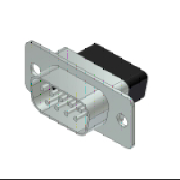
# Autodesk Inventor part: D-Sub Male 37CKT Crimp
Saved by Autodesk Inventor 2017 (Build 210142000, 142)
## iProperties
Created: 2016-02-22
Part Number: D-Sub Male 37CKT Crimp
Material: Générique
Description: Bouchon, Connecteur sous-miniature D
Document SubType Name: Modeling
Designer: Adrien MARY
Language: fr-FR
Size Designation: D-Sub Male Crimp 37CKT
Categories: <MemberInstance><Categories><Category DisplayName="Câble et faisceau" InternalName="e4a7e005-5e42-4d16-b293-125e7f0d0512" Mnemonic="CABLEANDHARNESS"><Category DisplayName="Raccords" InternalName="6f634eba-a678-4820-a31d-2c2d5ee6728e" Mnemonic="CONNECTORS"><CategoryParameter DisplayName="RefDes" InternalName="c3740e8c-60ab-4d5d-8584-52b73222f2f0" Mnemonic="REFDES"/><Category DisplayName="Fil discret" InternalName="9a3407de-09b2-4cdb-8c40-9708d5144a28" Mnemonic="DISCRETEWIRE"/></Category></Category><Category DisplayName="Type de données" InternalName="23b78d0f-2648-40c6-8793-ca6db495c9e8" Mnemonic="DATATYPE"><CategoryParameter DisplayName="AfficherNom" InternalName="05415f3d-3907-474b-a020-eb9d644f4cf3" Mnemonic="DISPLAYNAME"/><CategoryParameter DisplayName="Norme" InternalName="0c0a119c-1e12-4c84-803f-101930972f5e" Mnemonic="STANDARD"/><CategoryParameter DisplayName="Description" InternalName="13903e3d-64b1-4950-80da-f627842ea37f" Mnemonic="DESCRIPTION"/><CategoryParameter DisplayName="Désignation" InternalName="2675968c-4ce5-49e0-a4f5-552d29089031" Mnemonic="DESIGNATION"/><CategoryParameter DisplayName="Ligne par défaut" InternalName="2af9ec52-faaa-4026-b378-f9fa4afca842" Mnemonic="DEFAULTROW"/><CategoryParameter DisplayName="Nom de dossier" InternalName="3f06958e-8713-4116-9be7-ed6184ecc97b" Mnemonic="FOLDERNAME"/><CategoryParameter DisplayName="Guide révision" InternalName="45a75005-10b1-4dfc-8d6d-dfe629f0b93c" Mnemonic="REVISIONGUID"/><CategoryParameter DisplayName="NomFichier" InternalName="8b46a4cc-9585-4fed-90c3-899f57e09a73" Mnemonic="FILENAME"/><CategoryParameter DisplayName="OrgNorm" InternalName="8f5914e1-4693-403f-8ab5-d37768198c9d" Mnemonic="STDSORG"/><CategoryParameter DisplayName="Version de la famille" InternalName="914462f6-6e19-4b14-ba84-155b9680b1d0" Mnemonic="FAMILYREVISION"/><CategoryParameter DisplayName="Version standard" InternalName="91d5a463-65c2-4fde-b823-3b7fea5e8e17" Mnemonic="STANDARDREVISION"/><CategoryParameter DisplayName="Révision de membre" InternalName="a65d44b9-392f-4f4f-857b-e4b3d54996fe" Mnemonic="MEMBERREVISION"/><CategoryParameter DisplayName="DélimiterFormat" InternalName="bc51e27b-3422-4e78-93ef-cec197ddf230" Mnemonic="CLIPFORMAT"/><CategoryParameter DisplayName="Fabricant" InternalName="cd6c7a72-a28a-4e50-99a9-2c7f4e13e5ad" Mnemonic="MANUFACTURER"/><CategoryParameter DisplayName="NomInterne" InternalName="cf1d0246-76d9-4b4a-8305-fa0409afb5c1" Mnemonic="INTERNALNAME"/><CategoryParameter DisplayName="Métrique" InternalName="e2385c5b-1ea4-4823-96a8-8de651266ec3" Mnemonic="ISMETRIC"/><Category DisplayName="Pièce" InternalName="c0e0b642-3bcb-4cc8-9e80-f96d35c4afa4" Mnemonic="PART"><CategoryParameter DisplayName="Numéro de pièce" InternalName="016b6077-bfbe-49bd-92c9-d8d59c39c941" Mnemonic="PARTNUMBER"/><CategoryParameter DisplayName="Numéro de stock" InternalName="4dba7c1c-e26c-444e-836c-b08b433409a8" Mnemonic="STOCKNUMBER"/><CategoryParameter DisplayName="Clé matière" InternalName="5c9a8adb-dd2b-4535-b97f-0a94a95fe41f" Mnemonic="MATERIALKEY"/><CategoryParameter DisplayName="Matière" InternalName="818a152a-d3c3-49ca-80ee-df7d91421b8e" Mnemonic="MATERIAL"/></Category></Category></Categories><FamilyTemplate Id="D-Sub Male Crimp"><FamilyTemplateParameters><FamilyTemplateParameter ObjectType="kUserParameterObject" ValueType="xs:double" Id="1" ObjectReferenceKey="DimA"/><FamilyTemplateParameter ObjectType="kUserParameterObject" ValueType="xs:double" Id="2" ObjectReferenceKey="DimB"/><FamilyTemplateParameter ObjectType="kUserParameterObject" ValueType="xs:double" Id="3" ObjectReferenceKey="DimC"/><FamilyTemplateParameter ObjectType="kUserParameterObject" ValueType="xs:double" Id="4" ObjectReferenceKey="DimD"/><FamilyTemplateParameter ObjectType="kUserParameterObject" ValueType="xs:double" Id="5" ObjectReferenceKey="DimE"/><FamilyTemplateParameter ObjectType="kUserParameterObject" ValueType="xs:double" Id="6" ObjectReferenceKey="Holes_R1"/><FamilyTemplateParameter ObjectType="kUserParameterObject" ValueType="xs:double" Id="7" ObjectReferenceKey="Holes_R2"/><FamilyTemplateParameter ObjectType="kUserParameterObject" ValueType="xs:double" Id="8" ObjectReferenceKey="P10C"/><FamilyTemplateParameter ObjectType="kUserParameterObject" ValueType="xs:double" Id="9" ObjectReferenceKey="P10R"/><FamilyTemplateParameter ObjectType="kUserParameterObject" ValueType="xs:double" Id="10" ObjectReferenceKey="P11C"/><FamilyTemplateParameter ObjectType="kUserParameterObject" ValueType="xs:double" Id="11" ObjectReferenceKey="P11R"/><FamilyTemplateParameter ObjectType="kUserParameterObject" ValueType="xs:double" Id="12" ObjectReferenceKey="P12C"/><FamilyTemplateParameter ObjectType="kUserParameterObject" ValueType="xs:double" Id="13" ObjectReferenceKey="P12R"/><FamilyTemplateParameter ObjectType="kUserParameterObject" ValueType="xs:double" Id="14" ObjectReferenceKey="P13C"/><FamilyTemplateParameter ObjectType="kUserParameterObject" ValueType="xs:double" Id="15" ObjectReferenceKey="P13R"/><FamilyTemplateParameter ObjectType="kUserParameterObject" ValueType="xs:double" Id="16" ObjectReferenceKey="P14C"/><FamilyTemplateParameter ObjectType="kUserParameterObject" ValueType="xs:double" Id="17" ObjectReferenceKey="P14R"/><FamilyTemplateParameter ObjectType="kUserParameterObject" ValueType="xs:double" Id="18" ObjectReferenceKey="P15C"/><FamilyTemplateParameter ObjectType="kUserParameterObject" ValueType="xs:double" Id="19" ObjectReferenceKey="P15R"/><FamilyTemplateParameter ObjectType="kUserParameterObject" ValueType="xs:double" Id="20" ObjectReferenceKey="P16C"/><FamilyTemplateParameter ObjectType="kUserParameterObject" ValueType="xs:double" Id="21" ObjectReferenceKey="P16R"/><FamilyTemplateParameter ObjectType="kUserParameterObject" ValueType="xs:double" Id="22" ObjectReferenceKey="P17C"/><FamilyTemplateParameter ObjectType="kUserParameterObject" ValueType="xs:double" Id="23" ObjectReferenceKey="P17R"/><FamilyTemplateParameter ObjectType="kUserParameterObject" ValueType="xs:double" Id="24" ObjectReferenceKey="P18C"/><FamilyTemplateParameter ObjectType="kUserParameterObject" ValueType="xs:double" Id="25" ObjectReferenceKey="P18R"/><FamilyTemplateParameter ObjectType="kUserParameterObject" ValueType="xs:double" Id="26" ObjectReferenceKey="P19C"/><FamilyTemplateParameter ObjectType="kUserParameterObject" ValueType="xs:double" Id="27" ObjectReferenceKey="P19R"/><FamilyTemplateParameter ObjectType="kUserParameterObject" ValueType="xs:double" Id="28" ObjectReferenceKey="P20C"/><FamilyTemplateParameter ObjectType="kUserParameterObject" ValueType="xs:double" Id="29" ObjectReferenceKey="P20R"/><FamilyTemplateParameter ObjectType="kUserParameterObject" ValueType="xs:double" Id="30" ObjectReferenceKey="P21C"/><FamilyTemplateParameter ObjectType="kUserParameterObject" ValueType="xs:double" Id="31" ObjectReferenceKey="P21R"/><FamilyTemplateParameter ObjectType="kUserParameterObject" ValueType="xs:double" Id="32" ObjectReferenceKey="P22C"/><FamilyTemplateParameter ObjectType="kUserParameterObject" ValueType="xs:double" Id="33" ObjectReferenceKey="P22R"/><FamilyTemplateParameter ObjectType="kUserParameterObject" ValueType="xs:double" Id="34" ObjectReferenceKey="P23C"/><FamilyTemplateParameter ObjectType="kUserParameterObject" ValueType="xs:double" Id="35" ObjectReferenceKey="P23R"/><FamilyTemplateParameter ObjectType="kUserParameterObject" ValueType="xs:double" Id="36" ObjectReferenceKey="P24C"/><FamilyTemplateParameter ObjectType="kUserParameterObject" ValueType="xs:double" Id="37" ObjectReferenceKey="P24R"/><FamilyTemplateParameter ObjectType="kUserParameterObject" ValueType="xs:double" Id="38" ObjectReferenceKey="P25C"/><FamilyTemplateParameter ObjectType="kUserParameterObject" ValueType="xs:double" Id="39" ObjectReferenceKey="P25R"/><FamilyTemplateParameter ObjectType="kUserParameterObject" ValueType="xs:double" Id="40" ObjectReferenceKey="P26C"/><FamilyTemplateParameter ObjectType="kUserParameterObject" ValueType="xs:double" Id="41" ObjectReferenceKey="P26R"/><FamilyTemplateParameter ObjectType="kUserParameterObject" ValueType="xs:double" Id="42" ObjectReferenceKey="P27C"/><FamilyTemplateParameter ObjectType="kUserParameterObject" ValueType="xs:double" Id="43" ObjectReferenceKey="P27R"/><FamilyTemplateParameter ObjectType="kUserParameterObject" ValueType="xs:double" Id="44" ObjectReferenceKey="P28C"/><FamilyTemplateParameter ObjectType="kUserParameterObject" ValueType="xs:double" Id="45" ObjectReferenceKey="P28R"/><FamilyTemplateParameter ObjectType="kUserParameterObject" ValueType="xs:double" Id="46" ObjectReferenceKey="P29C"/><FamilyTemplateParameter ObjectType="kUserParameterObject" ValueType="xs:double" Id="47" ObjectReferenceKey="P29R"/><FamilyTemplateParameter ObjectType="kUserParameterObject" ValueType="xs:double" Id="48" ObjectReferenceKey="P30C"/><FamilyTemplateParameter ObjectType="kUserParameterObject" ValueType="xs:double" Id="49" ObjectReferenceKey="P30R"/><FamilyTemplateParameter ObjectType="kUserParameterObject" ValueType="xs:double" Id="50" ObjectReferenceKey="P31C"/><FamilyTemplateParameter ObjectType="kUserParameterObject" ValueType="xs:double" Id="51" ObjectReferenceKey="P31R"/><FamilyTemplateParameter ObjectType="kUserParameterObject" ValueType="xs:double" Id="52" ObjectReferenceKey="P32C"/><FamilyTemplateParameter ObjectType="kUserParameterObject" ValueType="xs:double" Id="53" ObjectReferenceKey="P32R"/><FamilyTemplateParameter ObjectType="kUserParameterObject" ValueType="xs:double" Id="54" ObjectReferenceKey="P33C"/><FamilyTemplateParameter ObjectType="kUserParameterObject" ValueType="xs:double" Id="55" ObjectReferenceKey="P33R"/><FamilyTemplateParameter ObjectType="kUserParameterObject" ValueType="xs:double" Id="56" ObjectReferenceKey="P34C"/><FamilyTemplateParameter ObjectType="kUserParameterObject" ValueType="xs:double" Id="57" ObjectReferenceKey="P34R"/><FamilyTemplateParameter ObjectType="kUserParameterObject" ValueType="xs:double" Id="58" ObjectReferenceKey="P35C"/><FamilyTemplateParameter ObjectType="kUserParameterObject" ValueType="xs:double" Id="59" ObjectReferenceKey="P35R"/><FamilyTemplateParameter ObjectType="kUserParameterObject" ValueType="xs:double" Id="60" ObjectReferenceKey="P36C"/><FamilyTemplateParameter ObjectType="kUserParameterObject" ValueType="xs:double" Id="61" ObjectReferenceKey="P36R"/><FamilyTemplateParameter ObjectType="kUserParameterObject" ValueType="xs:double" Id="62" ObjectReferenceKey="P37C"/><FamilyTemplateParameter ObjectType="kUserParameterObject" ValueType="xs:double" Id="63" ObjectReferenceKey="P6C"/><FamilyTemplateParameter ObjectType="kUserParameterObject" ValueType="xs:double" Id="64" ObjectReferenceKey="P6R"/><FamilyTemplateParameter ObjectType="kUserParameterObject" ValueType="xs:double" Id="65" ObjectReferenceKey="P7C"/><FamilyTemplateParameter ObjectType="kUserParameterObject" ValueType="xs:double" Id="66" ObjectReferenceKey="P7R"/><FamilyTemplateParameter ObjectType="kUserParameterObject" ValueType="xs:double" Id="67" ObjectReferenceKey="P8C"/><FamilyTemplateParameter ObjectType="kUserParameterObject" ValueType="xs:double" Id="68" ObjectReferenceKey="P8R"/><FamilyTemplateParameter ObjectType="kUserParameterObject" ValueType="xs:double" Id="69" ObjectReferenceKey="P9C"/><FamilyTemplateParameter ObjectType="kUserParameterObject" ValueType="xs:double" Id="70" ObjectReferenceKey="P9R"/><FamilyTemplateParameter ObjectType="kPropertyObject" ValueType="xs:string" Id="100" ObjectReferenceKey="{32853F0F-3444-11d1-9E93-0060B03C1CA6}" SubObjectId="52"/><FamilyTemplateParameter ObjectType="kPropertyObject" ValueType="xs:string" Id="105" ObjectReferenceKey="{32853F0F-3444-11d1-9E93-0060B03C1CA6}" SubObjectId="5"/><FamilyTemplateParameter ObjectType="kPartComponentDefinitionObject" ValueType="xs:string" Id="110" SubObjectId="Material"/><FamilyTemplateParameter ObjectType="kPartFeatureObject" ValueType="xs:boolean" Id="200" ObjectReferenceKey="10020000100000005cbc0200000000008000000000000000" SubObjectId="Suppressed"/><FamilyTemplateParameter ObjectType="kPartFeatureObject" ValueType="xs:boolean" Id="201" ObjectReferenceKey="100200001000000077bc0200000000008000000000000000" SubObjectId="Suppressed"/><FamilyTemplateParameter ObjectType="kPartFeatureObject" ValueType="xs:boolean" Id="202" ObjectReferenceKey="10020000100000007abc0200000000008000000000000000" SubObjectId="Suppressed"/><FamilyTemplateParameter ObjectType="kPartFeatureObject" ValueType="xs:boolean" Id="203" ObjectReferenceKey="10020000100000007dbc0200000000008000000000000000" SubObjectId="Suppressed"/><FamilyTemplateParameter ObjectType="kPartFeatureObject" ValueType="xs:boolean" Id="204" ObjectReferenceKey="100200001000000080bc0200000000008000000000000000" SubObjectId="Suppressed"/><FamilyTemplateParameter ObjectType="kPartFeatureObject" ValueType="xs:boolean" Id="205" ObjectReferenceKey="100200001000000083bc0200000000008000000000000000" SubObjectId="Suppressed"/><FamilyTemplateParameter ObjectType="kPartFeatureObject" ValueType="xs:boolean" Id="206" ObjectReferenceKey="100200001000000086bc0200000000008000000000000000" SubObjectId="Suppressed"/><FamilyTemplateParameter ObjectType="kPartFeatureObject" ValueType="xs:boolean" Id="207" ObjectReferenceKey="100200001000000089bc0200000000008000000000000000" SubObjectId="Suppressed"/><FamilyTemplateParameter ObjectType="kPartFeatureObject" ValueType="xs:boolean" Id="208" ObjectReferenceKey="10020000100000008cbc0200000000008000000000000000" SubObjectId="Suppressed"/><FamilyTemplateParameter ObjectType="kPartFeatureObject" ValueType="xs:boolean" Id="209" ObjectReferenceKey="10020000100000008fbc0200000000008000000000000000" SubObjectId="Suppressed"/><FamilyTemplateParameter ObjectType="kPartFeatureObject" ValueType="xs:boolean" Id="210" ObjectReferenceKey="100200001000000092bc0200000000008000000000000000" SubObjectId="Suppressed"/><FamilyTemplateParameter ObjectType="kPartFeatureObject" ValueType="xs:boolean" Id="211" ObjectReferenceKey="10020000100000005fbc0200000000008000000000000000" SubObjectId="Suppressed"/><FamilyTemplateParameter ObjectType="kPartFeatureObject" ValueType="xs:boolean" Id="212" ObjectReferenceKey="100200001000000095bc0200000000008000000000000000" SubObjectId="Suppressed"/><FamilyTemplateParameter ObjectType="kPartFeatureObject" ValueType="xs:boolean" Id="213" ObjectReferenceKey="100200001000000098bc0200000000008000000000000000" SubObjectId="Suppressed"/><FamilyTemplateParameter ObjectType="kPartFeatureObject" ValueType="xs:boolean" Id="214" ObjectReferenceKey="10020000100000009bbc0200000000008000000000000000" SubObjectId="Suppressed"/><FamilyTemplateParameter ObjectType="kPartFeatureObject" ValueType="xs:boolean" Id="215" ObjectReferenceKey="10020000100000009ebc0200000000008000000000000000" SubObjectId="Suppressed"/><FamilyTemplateParameter ObjectType="kPartFeatureObject" ValueType="xs:boolean" Id="216" ObjectReferenceKey="1002000010000000a1bc0200000000008000000000000000" SubObjectId="Suppressed"/><FamilyTemplateParameter ObjectType="kPartFeatureObject" ValueType="xs:boolean" Id="217" ObjectReferenceKey="1002000010000000a4bc0200000000008000000000000000" SubObjectId="Suppressed"/><FamilyTemplateParameter ObjectType="kPartFeatureObject" ValueType="xs:boolean" Id="218" ObjectReferenceKey="1002000010000000a7bc0200000000008000000000000000" SubObjectId="Suppressed"/><FamilyTemplateParameter ObjectType="kPartFeatureObject" ValueType="xs:boolean" Id="219" ObjectReferenceKey="1002000010000000aabc0200000000008000000000000000" SubObjectId="Suppressed"/><FamilyTemplateParameter ObjectType="kPartFeatureObject" ValueType="xs:boolean" Id="220" ObjectReferenceKey="1002000010000000adbc0200000000008000000000000000" SubObjectId="Suppressed"/><FamilyTemplateParameter ObjectType="kPartFeatureObject" ValueType="xs:boolean" Id="221" ObjectReferenceKey="1002000010000000b0bc0200000000008000000000000000" SubObjectId="Suppressed"/><FamilyTemplateParameter ObjectType="kPartFeatureObject" ValueType="xs:boolean" Id="222" ObjectReferenceKey="100200001000000062bc0200000000008000000000000000" SubObjectId="Suppressed"/><FamilyTemplateParameter ObjectType="kPartFeatureObject" ValueType="xs:boolean" Id="223" ObjectReferenceKey="1002000010000000b3bc0200000000008000000000000000" SubObjectId="Suppressed"/><FamilyTemplateParameter ObjectType="kPartFeatureObject" ValueType="xs:boolean" Id="224" ObjectReferenceKey="1002000010000000b6bc0200000000008000000000000000" SubObjectId="Suppressed"/><FamilyTemplateParameter ObjectType="kPartFeatureObject" ValueType="xs:boolean" Id="225" ObjectReferenceKey="1002000010000000b9bc0200000000008000000000000000" SubObjectId="Suppressed"/><FamilyTemplateParameter ObjectType="kPartFeatureObject" ValueType="xs:boolean" Id="226" ObjectReferenceKey="1002000010000000bcbc0200000000008000000000000000" SubObjectId="Suppressed"/><FamilyTemplateParameter ObjectType="kPartFeatureObject" ValueType="xs:boolean" Id="227" ObjectReferenceKey="1002000010000000bfbc0200000000008000000000000000" SubObjectId="Suppressed"/><FamilyTemplateParameter ObjectType="kPartFeatureObject" ValueType="xs:boolean" Id="228" ObjectReferenceKey="1002000010000000c2bc0200000000008000000000000000" SubObjectId="Suppressed"/><FamilyTemplateParameter ObjectType="kPartFeatureObject" ValueType="xs:boolean" Id="229" ObjectReferenceKey="1002000010000000c5bc0200000000008000000000000000" SubObjectId="Suppressed"/><FamilyTemplateParameter ObjectType="kPartFeatureObject" ValueType="xs:boolean" Id="230" ObjectReferenceKey="1002000010000000c8bc0200000000008000000000000000" SubObjectId="Suppressed"/><FamilyTemplateParameter ObjectType="kPartFeatureObject" ValueType="xs:boolean" Id="231" ObjectReferenceKey="100200001000000065bc0200000000008000000000000000" SubObjectId="Suppressed"/><FamilyTemplateParameter ObjectType="kPartFeatureObject" ValueType="xs:boolean" Id="232" ObjectReferenceKey="100200001000000068bc0200000000008000000000000000" SubObjectId="Suppressed"/><FamilyTemplateParameter ObjectType="kPartFeatureObject" ValueType="xs:boolean" Id="233" ObjectReferenceKey="10020000100000006bbc0200000000008000000000000000" SubObjectId="Suppressed"/><FamilyTemplateParameter ObjectType="kPartFeatureObject" ValueType="xs:boolean" Id="234" ObjectReferenceKey="10020000100000006ebc0200000000008000000000000000" SubObjectId="Suppressed"/><FamilyTemplateParameter ObjectType="kPartFeatureObject" ValueType="xs:boolean" Id="235" ObjectReferenceKey="100200001000000071bc0200000000008000000000000000" SubObjectId="Suppressed"/><FamilyTemplateParameter ObjectType="kPartFeatureObject" ValueType="xs:boolean" Id="236" ObjectReferenceKey="100200001000000074bc0200000000008000000000000000" SubObjectId="Suppressed"/></FamilyTemplateParameters></FamilyTemplate><CategoryParameterMap><ParamToTemplateMap><ParamToTemplate CategoryParameter="//CategoryParameter[@InternalName='05415f3d-3907-474b-a020-eb9d644f4cf3']" ConstantValue="D-Sub Male Crimp"/><ParamToTemplate CategoryParameter="//CategoryParameter[@InternalName='0c0a119c-1e12-4c84-803f-101930972f5e']" TemplateParameter="102"/><ParamToTemplate CategoryParameter="//CategoryParameter[@InternalName='13903e3d-64b1-4950-80da-f627842ea37f']" ConstantValue="Plug, Subminiature D Connector"/><ParamToTemplate CategoryParameter="//CategoryParameter[@InternalName='2af9ec52-faaa-4026-b378-f9fa4afca842']" ConstantValue="1"/><ParamToTemplate CategoryParameter="//CategoryParameter[@InternalName='3f06958e-8713-4116-9be7-ed6184ecc97b']" ConstantValue="D-Sub Male Crimp"/><ParamToTemplate CategoryParameter="//CategoryParameter[@InternalName='45a75005-10b1-4dfc-8d6d-dfe629f0b93c']" ConstantValue="6bfec97e-a90e-497f-8d9f-e40cc73ef834"/><ParamToTemplate CategoryParameter="//CategoryParameter[@InternalName='8f5914e1-4693-403f-8ab5-d37768198c9d']" TemplateParameter="101"/><ParamToTemplate CategoryParameter="//CategoryParameter[@InternalName='914462f6-6e19-4b14-ba84-155b9680b1d0']" ConstantValue="11"/><ParamToTemplate CategoryParameter="//CategoryParameter[@InternalName='91d5a463-65c2-4fde-b823-3b7fea5e8e17']" TemplateParameter="103"/><ParamToTemplate CategoryParameter="//CategoryParameter[@InternalName='bc51e27b-3422-4e78-93ef-cec197ddf230']" ConstantValue="CF_INVENTOR.STDPARTS"/><ParamToTemplate CategoryParameter="//CategoryParameter[@InternalName='cd6c7a72-a28a-4e50-99a9-2c7f4e13e5ad']" TemplateParameter="104"/><ParamToTemplate CategoryParameter="//CategoryParameter[@InternalName='cf1d0246-76d9-4b4a-8305-fa0409afb5c1']" ConstantValue="1b68272e-2c5e-46fd-a1a0-13114f04d71e"/><ParamToTemplate CategoryParameter="//CategoryParameter[@InternalName='e2385c5b-1ea4-4823-96a8-8de651266ec3']" ConstantValue="false"/><ParamToTemplate CategoryParameter="//CategoryParameter[@InternalName='8b46a4cc-9585-4fed-90c3-899f57e09a73']" ConstantValue="D-Sub Male Crimp 37CKT"/><ParamToTemplate CategoryParameter="//CategoryParameter[@InternalName='a65d44b9-392f-4f4f-857b-e4b3d54996fe']" ConstantValue="05c4e255-4499-4a76-b96a-0caab7a32f8d"/><ParamToTemplate CategoryParameter="//CategoryParameter[@InternalName='2675968c-4ce5-49e0-a4f5-552d29089031']" TemplateParameter="100"/><ParamToTemplate CategoryParameter="//CategoryParameter[@InternalName='818a152a-d3c3-49ca-80ee-df7d91421b8e']" TemplateParameter="110"/><ParamToTemplate CategoryParameter="//CategoryParameter[@InternalName='016b6077-bfbe-49bd-92c9-d8d59c39c941']" TemplateParameter="105"/></ParamToTemplateMap></CategoryParameterMap></MemberInstance>
Mass: 4.69725 g
Surface Area: 80.6213 cm^2
Volume: 4.69725 cm^3
Density: 1 g/cm^3
Appearance: Par défaut
GlobalPropertyList: <PropertyList/>
IsCustomPart: 0
Author: Adrien MARY
Autodesk Inventor part; units mm, degrees
ref_plane "YZ Plane" through (0, 0, 0) normal (1, 0, 0) x (0, 1, 0)
ref_plane "XZ Plane" through (0, 0, 0) normal (0, 1, 0) x (-1, 0, 0)
ref_plane "XY Plane" through (0, 0, 0) normal (0, 0, 1) x (1, 0, 0)
sketch "Sketch1" plane through (0, 0, 0) normal (0, 0, 1) x (1, 0, 0)
  circle A0 centre (-31.75, 0) radius 1.524
  circle A1 centre (31.75, 0) radius 1.524
  arc A2 (-33.0835, 6.2992) -> (-34.6583, 4.7244) centre (-33.0835, 4.7244) ccw
  line L0 (-34.6583, 4.7244) -> (-34.6583, -4.7244)
  arc A3 (-34.6583, -4.7244) -> (-33.0835, -6.2992) centre (-33.0835, -4.7244) ccw
  line L1 (-33.0835, -6.2992) -> (33.0835, -6.2992)
  arc A4 (33.0835, -6.2992) -> (34.6583, -4.7244) centre (33.0835, -4.7244) ccw
  line L2 (34.6583, -4.7244) -> (34.6583, 4.7244)
  arc A5 (34.6583, 4.7244) -> (33.0835, 6.2992) centre (33.0835, 4.7244) ccw
  line L3 (33.0835, 6.2992) -> (-33.0835, 6.2992)
  line L4 (0, 6.2992) -> (0, -6.2992) construction
  line L5 (-31.75, 0) -> (31.75, 0) construction
  line L6 (34.6583, 4.7244) -> (33.0835, 4.7244) construction
  line L7 (33.0835, 4.7244) -> (33.0835, 6.2992) construction
  line L8 (34.6583, -4.7244) -> (33.0835, -4.7244) construction
  line L9 (33.0835, -4.7244) -> (33.0835, -6.2992) construction
  line L10 (-33.0835, 6.2992) -> (-33.0835, 4.7244) construction
  line L11 (-33.0835, 4.7244) -> (-34.6583, 4.7244) construction
  line L12 (-34.6583, -4.7244) -> (-33.0835, -4.7244) construction
  line L13 (-33.0835, -4.7244) -> (-33.0835, -6.2992) construction
  point P0 (0, 0)
  point P1 (-34.6583, 0)
  point P2 (34.6583, 0)
  point P3 (0, 0)
  point P4 (0, 0)
  point P5 (33.0835, 5.5118)
  point P6 (33.0835, -5.5118)
  dimension "d124" = 69.3166
  dimension "d125" = 12.5984
  dimension "d126" = 1.5748
  dimension "d134" = 3.048
  dimension "d135" = 63.5
  constraints: 28 end point, 8 point on circle, 6 centre point, 6 midpoint, 5 perpendicular, 4 horizontal alignment, 4 vertical alignment, 3 equal radius, 3 parallel, 1 coincident
  measures "d124" distance between parallel lines of L2 L0
  measures "d125" distance between parallel lines of L1 L3
  measures "d126" radius of A5
  measures "d134" diameter of A0
  measures "d135" distance of L5.start L5.end
extrude "Extrusion1" add sketch "Sketch1" against normal mid plane 0.762
sketch "Sketch2" plane through (0, 0, 0.381) normal (0, 0, 1) x (1, 0, 0)
  line L0 (-33.0835, 6.2992) -> (33.0835, 6.2992) projected
  line L1 (33.0835, -6.2992) -> (-33.0835, -6.2992) projected
  arc A0 (-24.8793, 3.9497) -> (-27.3807, 0.9686) centre (-24.8793, 1.4097) ccw
  line L2 (-27.3807, 0.9686) -> (-26.8836, -1.8508)
  arc A1 (-26.8836, -1.8508) -> (-24.3822, -3.9497) centre (-24.3822, -1.4097) ccw
  line L3 (-24.3822, -3.9497) -> (24.3822, -3.9497)
  arc A2 (24.3822, -3.9497) -> (26.8836, -1.8508) centre (24.3822, -1.4097) ccw
  line L4 (26.8836, -1.8508) -> (27.3807, 0.9686)
  arc A3 (27.3807, 0.9686) -> (24.8793, 3.9497) centre (24.8793, 1.4097) ccw
  line L5 (24.8793, 3.9497) -> (-24.8793, 3.9497)
  line L6 (0, 3.9497) -> (0, -3.9497) construction
  line L7 (-27.4193, 6.2992) -> (-27.4193, -6.2992) construction
  line L8 (27.4193, 6.2992) -> (27.4193, -6.2992) construction
  line L9 (34.6583, 4.7244) -> (34.6583, -4.7244) projected
  arc A4 (-24.8793, 4.3561) -> (-27.7809, 0.8981) centre (-24.8793, 1.4097) ccw
  line L10 (-24.8793, 4.3561) -> (24.8793, 4.3561)
  line L11 (-24.3822, -4.3561) -> (24.3822, -4.3561)
  arc A5 (24.3822, -4.3561) -> (27.2838, -1.9213) centre (24.3822, -1.4097) ccw
  line L12 (-27.7809, 0.8981) -> (-27.2838, -1.9213)
  line L13 (27.7809, 0.8981) -> (27.2838, -1.9213)
  arc A6 (27.7809, 0.8981) -> (24.8793, 4.3561) centre (24.8793, 1.4097) ccw
  arc A7 (-27.2838, -1.9213) -> (-24.3822, -4.3561) centre (-24.3822, -1.4097) ccw
  point P0 (0, 6.2738)
  point P1 (34.6583, 0)
  point P2 (0, 6.2992)
  point P3 (-34.6583, 0)
  point P4 (0, 0)
  point P5 (0, 6.2992)
  point P6 (34.6583, 0)
  dimension "d127" = 2.54
  dimension "d129" = 7.8994
  dimension "d131" = 10
  dimension "d132" = 10
  dimension "d133" = 54.8386
  dimension "d198" = 0.4971
  dimension "d199" = 2.8194
  dimension "d200" = 0.4971
  dimension "d201" = 2.8194
  dimension "d292" = 0.4064
  dimension "d293" = 0.4064
  dimension "d294" = 0.4064
  constraints: 22 end point, 16 point on circle, 8 centre point, 7 tangent, 6 midpoint, 4 coincident, 4 point on line, 3 equal radius, 3 parallel, 3 perpendicular, 2 vertical alignment, 1 horizontal alignment
  measures "d127" radius of A3
  measures "d129" distance between parallel lines of L3 L5
  measures "d131" angle of L6 L2
  measures "d132" angle of L4 L6
  measures "d133" distance between parallel lines of L8 L7
  measures "d198" horizontal distance of A1.centre A0.centre
  measures "d199" vertical distance of A1.centre A0.centre
  measures "d200" horizontal distance of A2.centre A3.centre
  measures "d201" vertical distance of A2.centre A3.centre
  measures "d292" radial gap between concentric circles of A0 A4
  measures "d293" distance between parallel lines of L10 L5
  measures "d294" distance between parallel lines of L3 L11
extrude "Extrusion2" add sketch "Sketch2" along normal blind 5.5372
sketch "Sketch3" plane through (0, 0, -0.381) normal (0, 0, -1) x (-1, 0, 0)
  arc A0 (-27.3779, 5.4991) -> (-28.9288, 3.6508) centre (-27.3779, 3.9243) ccw
  line L0 (-28.9288, 3.6508) -> (-27.5449, -4.1978)
  arc A1 (-27.5449, -4.1978) -> (-25.994, -5.4991) centre (-25.994, -3.9243) ccw
  line L1 (-25.994, -5.4991) -> (25.994, -5.4991)
  arc A2 (25.994, -5.4991) -> (27.5449, -4.1978) centre (25.994, -3.9243) ccw
  line L2 (27.5449, -4.1978) -> (28.9043, 3.5119)
  arc A3 (28.9043, 3.5119) -> (27.3779, 5.4991) centre (27.3845, 3.9243) ccw
  line L3 (27.3779, 5.4991) -> (-27.3779, 5.4991)
  line L4 (0, 5.4991) -> (0, -5.4991) construction
  line L5 (-28.9527, 6.2738) -> (-28.9527, -6.2738) construction
  line L6 (28.9593, 6.2738) -> (28.9593, -6.2738) construction
  line L7 (-33.0835, 6.2992) -> (33.0835, 6.2992) projected
  line L8 (-34.6583, -4.7244) -> (-34.6583, 4.7244) projected
  line L9 (33.0835, -6.2992) -> (-33.0835, -6.2992) projected
  line L10 (-27.3779, 5.4991) -> (-27.3779, 3.9243) construction
  line L11 (-27.3779, 3.9243) -> (-28.9288, 3.6508) construction
  line L12 (-27.5449, -4.1978) -> (-25.994, -3.9243) construction
  line L13 (-25.994, -3.9243) -> (-25.994, -5.4991) construction
  line L14 (25.994, -3.9243) -> (25.994, -5.4991) construction
  line L15 (25.994, -3.9243) -> (27.5449, -4.1978) construction
  line L16 (27.3779, 5.4991) -> (27.3845, 3.9243) construction
  line L17 (27.3845, 3.9243) -> (28.9043, 3.5119) construction
  line L18 (34.6583, 4.7244) -> (34.6583, -4.7244) projected
  point P0 (0, 0)
  point P1 (0, -6.2738)
  point P2 (34.6583, 0)
  point P3 (0, 6.2992)
  point P4 (-34.6583, 0)
  dimension "d114" = 10.9982
  dimension "d119" = 1.5748
  dimension "d120" = 10
  dimension "d121" = 10
  dimension "d122" = 57.912
  dimension "d204" = 90
  dimension "d205" = 100
  dimension "d206" = 90
  dimension "d207" = 80
  dimension "d208" = 90
  dimension "d209" = 80
  dimension "d210" = 105.42
  dimension "d211" = 90.238
  dimension "d295" = 1.3839
  dimension "d296" = 1.3905
  constraints: 30 end point, 8 point on circle, 5 midpoint, 4 centre point, 4 parallel, 3 equal radius, 3 perpendicular, 2 horizontal alignment, 2 tangent, 2 vertical alignment
  measures "d114" distance between parallel lines of L1 L3
  measures "d119" radius of A3
  measures "d120" angle of L4 L0
  measures "d121" angle of L2 L4
  measures "d122" distance between parallel lines of L6 L5
  measures "d204" angle of L3 L10
  measures "d205" angle of L10 L11
  measures "d206" angle of L1 L13
  measures "d207" angle of L13 L12
  measures "d208" angle of L1 L14
  measures "d209" angle of L15 L14
  measures "d210" angle of L16 L17
  measures "d211" angle of L3 L16
  measures "d295" horizontal distance of L12.end L10.end
  measures "d296" horizontal distance of L14.start L16.end
extrude "Extrusion3" add sketch "Sketch3" along normal blind 3.937
sketch "Sketch4" plane through (0, 0, -4.318) normal (0, 0, -1) x (-1, 0, 0)
  line L0 (-27.3779, 5.4991) -> (27.3779, 5.4991) projected
  arc A0 (-25.8953, 3.5814) -> (-27.096, 2.1505) centre (-25.8953, 2.3622) ccw
  line L1 (-27.096, 2.1505) -> (-26.2629, -2.5739)
  arc A1 (-26.2629, -2.5739) -> (-25.0623, -3.5814) centre (-25.0623, -2.3622) ccw
  line L2 (-25.0623, -3.5814) -> (25.0623, -3.5814)
  arc A2 (25.0623, -3.5814) -> (26.2629, -2.5739) centre (25.0623, -2.3622) ccw
  line L3 (26.2629, -2.5739) -> (27.096, 2.1505)
  arc A3 (27.096, 2.1505) -> (25.8953, 3.5814) centre (25.8953, 2.3622) ccw
  line L4 (25.8953, 3.5814) -> (-25.8953, 3.5814)
  line L5 (0, 3.5814) -> (0, -3.5814) construction
  circle A4 centre (-31.75, 0) radius 1.524 projected
  circle A5 centre (31.75, 0) radius 1.524 projected
  line L6 (34.6583, 4.7244) -> (34.6583, -4.7244) projected
  arc A6 (34.6583, 4.7244) -> (33.0835, 6.2992) centre (33.0835, 4.7244) ccw projected
  line L7 (-33.0835, 6.2992) -> (33.0835, 6.2992) projected
  arc A7 (-33.0835, 6.2992) -> (-34.6583, 4.7244) centre (-33.0835, 4.7244) ccw projected
  line L8 (-34.6583, -4.7244) -> (-34.6583, 4.7244) projected
  arc A8 (-34.6583, -4.7244) -> (-33.0835, -6.2992) centre (-33.0835, -4.7244) ccw projected
  line L9 (33.0835, -6.2992) -> (-33.0835, -6.2992) projected
  arc A9 (33.0835, -6.2992) -> (34.6583, -4.7244) centre (33.0835, -4.7244) ccw projected
  line L10 (-27.1145, 6.2992) -> (-27.1145, -6.2992) construction
  line L11 (27.1145, 6.2992) -> (27.1145, -6.2992) construction
  line L12 (-27.5449, -4.1978) -> (-28.9288, 3.6508) projected
  line L13 (25.994, -5.4991) -> (-25.994, -5.4991) projected
  line L14 (-25.8953, 2.3622) -> (-25.8953, 3.5814) construction
  line L15 (-25.8953, 2.3622) -> (-27.096, 2.1505) construction
  line L16 (-25.0623, -2.3622) -> (-25.0623, -3.5814) construction
  line L17 (-25.0623, -2.3622) -> (-26.2629, -2.5739) construction
  line L18 (25.0623, -2.3622) -> (26.2629, -2.5739) construction
  line L19 (25.0623, -2.3622) -> (25.0623, -3.5814) construction
  line L20 (25.8953, 3.5814) -> (25.8953, 2.3622) construction
  line L21 (25.8953, 2.3622) -> (27.096, 2.1505) construction
  point P0 (0, 0)
  point P1 (0, 5.4991)
  point P2 (-31.75, 0)
  dimension "d136" = 7.1628
  dimension "d137" = 1.2192
  dimension "d139" = 10
  dimension "d140" = 10
  dimension "d141" = 54.229
  dimension "d212" = 90
  dimension "d213" = 100
  dimension "d214" = 90
  dimension "d215" = 80
  dimension "d216" = 90
  dimension "d217" = 80
  dimension "d218" = 90
  dimension "d219" = 100
  constraints: 30 end point, 8 point on circle, 6 parallel, 5 perpendicular, 4 centre point, 4 midpoint, 4 point on line, 3 equal radius, 2 tangent, 1 horizontal alignment, 1 vertical alignment
  measures "d136" distance between parallel lines of L2 L4
  measures "d137" radius of A3
  measures "d139" angle of L5 L1
  measures "d140" angle of L3 L5
  measures "d141" distance between parallel lines of L11 L10
  measures "d212" angle of L4 L14
  measures "d213" angle of L15 L14
  measures "d214" angle of L2 L16
  measures "d215" angle of L16 L17
  measures "d216" angle of L2 L19
  measures "d217" angle of L18 L19
  measures "d218" angle of L4 L20
  measures "d219" angle of L21 L20
extrude "Extrusion4" add sketch "Sketch4" along normal blind 7.1882 contours L4 A3 L3 A2 L2 A1 L1 A0
sketch "Sketch14" plane through (0, 0, -11.5062) normal (0, 0, -1) x (-1, 0, 0)
  circle A0 centre (24.8285, 1.4224) radius 1.1049
  circle A1 centre (23.4621, -1.4224) radius 1.1049
  line L0 (24.8761, 3.4036) -> (24.8761, 2.6416)
  line L1 (24.8761, 2.6416) -> (24.7809, 2.6416)
  line L2 (24.7809, 2.6416) -> (24.7809, 3.2739)
  line L3 (24.7809, 3.2739) -> (24.6856, 3.1604)
  line L4 (24.6856, 3.1604) -> (24.6856, 3.2901)
  line L5 (24.6856, 3.2901) -> (24.7809, 3.4036)
  line L6 (24.7809, 3.4036) -> (24.8761, 3.4036)
  arc A2 (25.0623, -3.5814) -> (26.2629, -2.5739) centre (25.0623, -2.3622) ccw projected
  arc A3 (27.096, 2.1505) -> (25.8953, 3.5814) centre (25.8953, 2.3622) ccw projected
  point P0 (24.8285, 2.6416)
  dimension "d144" = 2.2098
  dimension "d162" = 2.2098
  dimension "d181" = 0.0953
  dimension "d182" = 40.006
  dimension "d183" = 0.1297
  dimension "d184" = 0.0953
  dimension "d185" = 0.762
  dimension "d186" = 0.6323
  dimension "d187" = 0.1482
  dimension "d188" = 0.1482
  dimension "d189" = 40.006
  dimension "d190" = 139.994
  dimension "d297" = 1.0668
  dimension "d298" = 0.9398
  dimension "d299" = 1.6002
  dimension "d300" = 0.9398
  constraints: 14 end point, 2 centre point, 1 midpoint, 1 vertical alignment
  measures "d144" diameter of A0
  measures "d162" diameter of A1
  measures "d181" distance of L0.end L1.end
  measures "d182" angle of L2 L3
  measures "d183" distance of L4.start L4.end
  measures "d184" distance of L6.start L0.start
  measures "d185" distance of L0.start L0.end
  measures "d186" distance of L1.end L2.end
  measures "d187" distance of L4.end L6.start
  measures "d188" distance of L2.end L4.start
  measures "d189" angle of L4 L3
  measures "d190" angle of L4 L5
  measures "d297" horizontal distance of A3.centre A0.centre
  measures "d298" vertical distance of A0.centre A3.centre
  measures "d299" horizontal distance of A2.centre A1.centre
  measures "d300" vertical distance of A2.centre A1.centre
extrude "Extrusion15" cut sketch "Sketch14" against normal up to surface (11.1252 mm away) contours A0
sketch "Sketch15" plane through (0, 0, 0.381) normal (0, 0, 1) x (1, 0, 0)
  arc A0 (27.3807, 0.9686) -> (24.8793, 3.9497) centre (24.8793, 1.4097) ccw
  circle A1 centre (-24.8412, 1.4224) radius 0.5334
  arc A2 (24.3822, -3.9497) -> (26.8836, -1.8508) centre (24.3822, -1.4097) ccw
  circle A3 centre (-23.4696, -1.4224) radius 0.5334
  arc A4 (-24.8793, 3.9497) -> (-27.3807, 0.9686) centre (-24.8793, 1.4097) ccw projected
  arc A5 (-26.8836, -1.8508) -> (-24.3822, -3.9497) centre (-24.3822, -1.4097) ccw projected
  dimension "d149" = 1.0668
  dimension "d301" = 0.0381
  dimension "d302" = 0.0127
  dimension "d303" = 0.9126
  dimension "d304" = 0.0127
  constraints: 4 centre point, 4 point on circle, 1 equal radius
  measures "d149" diameter of A1
  measures "d301" horizontal distance of A4.centre A1.centre
  measures "d302" vertical distance of A4.centre A1.centre
  measures "d303" horizontal distance of A5.centre A3.centre
  measures "d304" vertical distance of A5.centre A3.centre
extrude "Extrusion16" add sketch "Sketch15" along normal blind 5.08 contours A1
pattern_linear "Réseau rectangulaire7" count 19 spacing 2.7432 along (1, 0, 0) of "Extrusion15", "Extrusion16"
extrude "Extrusion17" cut sketch "Sketch14" against normal up to surface (11.1252 mm away) contours A1
extrude "Extrusion18" add sketch "Sketch15" along normal blind 5.08 contours A3
pattern_linear "Réseau rectangulaire8" count 18 spacing 2.7432 along (1, 0, 0) of "Extrusion17", "Extrusion18"
extrude "Extrusion19" add sketch "Sketch14" along normal blind 0.0254 contours L0 L1 L2 L3 L4 L5 L6
sketch "Sketch16" plane through (0, 0, -11.5062) normal (0, 0, -1) x (-1, 0, 0)
  arc A0 (-25.8953, 3.5814) -> (-27.096, 2.1505) centre (-25.8953, 2.3622) ccw projected
  line L0 (24.8761, 2.6416) -> (24.7809, 2.6416) projected
  line L1 (24.7809, 2.6416) -> (24.7809, 3.2739) projected
  line L2 (24.7809, 3.2739) -> (24.6856, 3.1604) projected
  line L3 (24.6856, 3.1604) -> (24.6856, 3.2901) projected
  line L4 (24.6856, 3.2901) -> (24.7809, 3.4036) projected
  line L5 (24.7809, 3.4036) -> (24.8761, 3.4036) projected
  line L6 (24.8761, 3.4036) -> (24.8761, 2.6416) projected
  line L7 (25.0623, -3.5814) -> (-25.0623, -3.5814) projected
  arc A1 (25.0623, -3.5814) -> (26.2629, -2.5739) centre (25.0623, -2.3622) ccw projected
  line L8 (27.096, 2.1505) -> (26.2629, -2.5739) projected
  arc A2 (27.096, 2.1505) -> (25.8953, 3.5814) centre (25.8953, 2.3622) ccw projected
  line L9 (-25.8953, 3.5814) -> (25.8953, 3.5814) projected
  line L10 (-26.2629, -2.5739) -> (-27.096, 2.1505) projected
  arc A3 (-26.2629, -2.5739) -> (-25.0623, -3.5814) centre (-25.0623, -2.3622) ccw projected
  line L11 (25.0623, -3.5814) -> (-25.0623, -3.5814) projected
  arc A4 (25.0623, -3.5814) -> (26.2629, -2.5739) centre (25.0623, -2.3622) ccw projected
  line L12 (27.096, 2.1505) -> (26.2629, -2.5739) projected
  arc A5 (27.096, 2.1505) -> (25.8953, 3.5814) centre (25.8953, 2.3622) ccw projected
  line L13 (-25.8953, 3.5814) -> (25.8953, 3.5814) projected
  line L14 (-26.2629, -2.5739) -> (-27.096, 2.1505) projected
  arc A6 (-26.2629, -2.5739) -> (-25.0623, -3.5814) centre (-25.0623, -2.3622) ccw projected
  point P0 (24.8285, 1.4224)
  point P1 (22.0853, 1.4224)
  point P2 (19.3421, 1.4224)
  point P3 (16.5989, 1.4224)
  point P4 (13.8557, 1.4224)
  point P5 (11.1125, 1.4224)
  point P6 (8.3693, 1.4224)
  point P7 (5.6261, 1.4224)
  point P8 (2.8829, 1.4224)
  point P9 (0.1397, 1.4224)
  point P10 (-2.6035, 1.4224)
  point P11 (-5.3467, 1.4224)
  point P12 (-8.0899, 1.4224)
  point P13 (-10.8331, 1.4224)
  point P14 (-13.5763, 1.4224)
  point P15 (-16.3195, 1.4224)
  point P16 (-19.0627, 1.4224)
  point P17 (-21.8059, 1.4224)
  point P18 (-24.5491, 1.4224)
  point P19 (-23.1775, -1.4224)
  point P20 (-20.4343, -1.4224)
  point P21 (-17.6911, -1.4224)
  point P22 (-14.9479, -1.4224)
  point P23 (-12.2047, -1.4224)
  point P24 (-9.5631, -1.4224)
  point P25 (-6.7183, -1.4224)
  point P26 (-3.9751, -1.4224)
  point P27 (-1.2319, -1.4224)
  point P28 (1.5113, -1.4224)
  point P29 (4.2545, -1.4224)
  point P30 (6.9977, -1.4224)
  point P31 (9.7409, -1.4224)
  point P32 (12.4841, -1.4224)
  point P33 (15.2273, -1.4224)
  point P34 (17.9705, -1.4224)
  point P35 (20.7137, -1.4224)
  point P36 (23.4569, -1.4224)
  dimension "P1C" = 1.0668
  dimension "P1R" = 0.9398
  dimension "P2C" = 3.81
  dimension "P2R" = 0.9398
  dimension "P3C" = 6.5532
  dimension "P3R" = 0.9398
  dimension "P4C" = 9.2964
  dimension "P4R" = 0.9398
  dimension "P5C" = 12.0396
  dimension "P5R" = 0.9398
  dimension "P6C" = 14.7828
  dimension "P6R" = 0.9398
  dimension "P7C" = 17.526
  dimension "P7R" = 0.9398
  dimension "P8C" = 20.2692
  dimension "P8R" = 0.9398
  dimension "P9C" = 23.0124
  dimension "P9R" = 0.9398
  dimension "P10C" = 25.7556
  dimension "P10R" = 0.9398
  dimension "P11C" = 28.4988
  dimension "P11R" = 0.9398
  dimension "P12C" = 31.242
  dimension "P12R" = 0.9398
  dimension "P13C" = 33.9852
  dimension "P13R" = 0.9398
  dimension "P14C" = 36.7284
  dimension "P14R" = 0.9398
  dimension "P15C" = 39.4716
  dimension "P15R" = 0.9398
  dimension "P16C" = 42.2148
  dimension "P16R" = 0.9398
  dimension "P17C" = 44.958
  dimension "P17R" = 0.9398
  dimension "P18C" = 47.7012
  dimension "P18R" = 0.9398
  dimension "P19C" = 50.4444
  dimension "P19R" = 0.9398
  dimension "P20C" = 2.4384
  dimension "P20R" = 3.7846
  dimension "P21C" = 5.1816
  dimension "P21R" = 3.7846
  dimension "P22C" = 7.9248
  dimension "P22R" = 3.7846
  dimension "P23C" = 10.668
  dimension "P23R" = 3.7846
  dimension "P24C" = 13.4112
  dimension "P24R" = 3.7846
  dimension "P25C" = 16.1544
  dimension "P25R" = 3.7846
  dimension "P26C" = 18.8976
  dimension "P26R" = 3.7846
  dimension "P27C" = 21.6408
  dimension "P27R" = 3.7846
  dimension "P28C" = 24.384
  dimension "P28R" = 3.7846
  dimension "P29C" = 27.1272
  dimension "P29R" = 3.7846
  dimension "P30C" = 29.8704
  dimension "P30R" = 3.7846
  dimension "P31C" = 32.6136
  dimension "P31R" = 3.7846
  dimension "P32C" = 35.4584
  dimension "P32R" = 3.7846
  measures "P1C" horizontal distance of A2.centre point (24.828, 1.422)
  measures "P1R" vertical distance of A2.centre point (24.828, 1.422)
  measures "P2C" horizontal distance of A2.centre point (22.085, 1.422)
  measures "P2R" vertical distance of A2.centre point (22.085, 1.422)
  measures "P3C" horizontal distance of A5.centre point (19.342, 1.422)
  measures "P3R" vertical distance of A2.centre point (19.342, 1.422)
  measures "P4C" horizontal distance of A5.centre point (16.599, 1.422)
  measures "P4R" vertical distance of A2.centre point (16.599, 1.422)
  measures "P5C" horizontal distance of A2.centre point (13.856, 1.422)
  measures "P5R" vertical distance of A5.centre point (13.856, 1.422)
  measures "P6C" horizontal distance of A2.centre point (11.112, 1.422)
  measures "P6R" vertical distance of A2.centre point (11.112, 1.422)
  measures "P7C" horizontal distance of A2.centre point (8.369, 1.422)
  measures "P7R" vertical distance of A2.centre point (8.369, 1.422)
  measures "P8C" horizontal distance of A2.centre point (5.626, 1.422)
  measures "P8R" vertical distance of A2.centre point (5.626, 1.422)
  measures "P9C" horizontal distance of A5.centre point (2.883, 1.422)
  measures "P9R" vertical distance of A2.centre point (2.883, 1.422)
  measures "P10C" horizontal distance of A5.centre point (0.14, 1.422)
  measures "P10R" vertical distance of A2.centre point (0.14, 1.422)
  measures "P11C" horizontal distance of A5.centre point (-2.604, 1.422)
  measures "P11R" vertical distance of A2.centre point (-2.604, 1.422)
  measures "P12C" horizontal distance of A2.centre point (-5.347, 1.422)
  measures "P12R" vertical distance of A2.centre point (-5.347, 1.422)
  measures "P13C" horizontal distance of A2.centre point (-8.09, 1.422)
  measures "P13R" vertical distance of A2.centre point (-8.09, 1.422)
  measures "P14C" horizontal distance of A2.centre point (-10.833, 1.422)
  measures "P14R" vertical distance of A2.centre point (-10.833, 1.422)
  measures "P15C" horizontal distance of A2.centre point (-13.576, 1.422)
  measures "P15R" vertical distance of A2.centre point (-13.576, 1.422)
  measures "P16C" horizontal distance of A2.centre point (-16.32, 1.422)
  measures "P16R" vertical distance of A2.centre point (-16.32, 1.422)
  measures "P17C" horizontal distance of A2.centre point (-19.063, 1.422)
  measures "P17R" vertical distance of A2.centre point (-19.063, 1.422)
  measures "P18C" horizontal distance of A2.centre point (-21.806, 1.422)
  measures "P18R" vertical distance of A5.centre point (-21.806, 1.422)
  measures "P19C" horizontal distance of A2.centre point (-24.549, 1.422)
  measures "P19R" vertical distance of A2.centre point (-24.549, 1.422)
  measures "P20C" horizontal distance of point (23.457, -1.422) A2.centre
  measures "P20R" vertical distance of A2.centre point (23.457, -1.422)
  measures "P21C" horizontal distance of A5.centre point (20.714, -1.422)
  measures "P21R" vertical distance of A2.centre point (20.714, -1.422)
  measures "P22C" horizontal distance of A2.centre point (17.97, -1.422)
  measures "P22R" vertical distance of A2.centre point (17.97, -1.422)
  measures "P23C" horizontal distance of A2.centre point (15.227, -1.422)
  measures "P23R" vertical distance of A2.centre point (15.227, -1.422)
  measures "P24C" horizontal distance of A2.centre point (12.484, -1.422)
  measures "P24R" vertical distance of A2.centre point (12.484, -1.422)
  measures "P25C" horizontal distance of A5.centre point (9.741, -1.422)
  measures "P25R" vertical distance of A2.centre point (9.741, -1.422)
  measures "P26C" horizontal distance of A2.centre point (6.998, -1.422)
  measures "P26R" vertical distance of A2.centre point (6.998, -1.422)
  measures "P27C" horizontal distance of A2.centre point (4.254, -1.422)
  measures "P27R" vertical distance of A2.centre point (4.254, -1.422)
  measures "P28C" horizontal distance of A2.centre point (1.511, -1.422)
  measures "P28R" vertical distance of A2.centre point (1.511, -1.422)
  measures "P29C" horizontal distance of A2.centre point (-1.232, -1.422)
  measures "P29R" vertical distance of A2.centre point (-1.232, -1.422)
  measures "P30C" horizontal distance of A2.centre point (-3.975, -1.422)
  measures "P30R" vertical distance of A2.centre point (-3.975, -1.422)
  measures "P31C" horizontal distance of A2.centre point (-6.718, -1.422)
  measures "P31R" vertical distance of A2.centre point (-6.718, -1.422)
  measures "P32C" horizontal distance of A2.centre point (-9.563, -1.422)
  measures "P32R" vertical distance of A2.centre point (-9.563, -1.422)
equation "\"DimA\" = 69.3166"
equation "\"DimB\" = 63.5"
equation "\"DimC\" = 54.8386"
equation "\"DimD\" = 57.912"
equation "\"DimE\" = 54.229"
equation "\"PinPitch\" = 2.7432"
body "Solid1"
